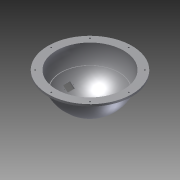
# Autodesk Inventor part: harvey_ballCup_ADNS9800_Vers1_1
Saved by Autodesk Inventor 2016 (Build 200138000, 138)
## iProperties
Created: 2012-05-12
Part Number: harvey_ballCup_ADNS9800_Vers1_1
Material: Generic
Document SubType Name: Modeling
Designer: charvey
Density: 1 g/cm^3
Appearance: Default
Author: charvey
Autodesk Inventor part; units mm, degrees
sketch "Sketch1" plane through (0, 0, 0) normal (0, 0, 1) x (1, 0, 0)
  arc A0 (0, -1.5875) -> (103.1875, 101.6) centre (0, 101.6) ccw
  arc A1 (0, -4.7625) -> (106.3625, 101.6) centre (0, 101.6) ccw
  line L0 (0, -1.5875) -> (0, -4.7625)
  line L1 (128.5875, 101.6) -> (128.5875, 95.25)
  line L2 (128.5875, 95.25) -> (106.1728, 95.25)
  line L3 (103.1875, 101.6) -> (128.5875, 101.6)
  arc A2 (0, 0) -> (87.9882, 50.8) centre (0, 101.6) ccw
  line L4 (87.9882, 50.8) -> (89.8166, 50.8)
  line L5 (0, 0) -> (0, -1.5875)
  dimension "d0" = 101.6
  dimension "d1" = 103.1875
  dimension "d2" = 106.3625
  dimension "d3" = 25.4
  dimension "d4" = 6.35
  dimension "d11" = 50.8
  constraints: 12 end point, 8 point on circle, 3 centre point, 2 coincident, 2 horizontal alignment, 2 parallel, 2 perpendicular, 1 point on line, 1 vertical
  measures "d0" distance of L5.start A0.centre
  measures "d1" distance of L0.start A0.centre
  measures "d2" distance of L0.end A1.centre
  measures "d3" distance of L3.start L1.start
  measures "d4" distance of L1.start L1.end
  measures "d11" vertical distance of L5.start L4.start
revolve "Revolution3" add sketch "Sketch1" angle 360 about axis through (0, -1.5875, 0) along (0, -1, 0)
ref_plane "Work Plane1" through (0, 127, 0) normal (0, 1, 0) x (-1, 0, 0)
sketch "Sketch4" plane through (0, 127, 0) normal (0, 1, 0) x (-1, 0, 0)
  line L0 (0, 0) -> (-141.4138, 0)
  line L1 (-141.4138, 0) -> (-141.4138, -141.6884)
  line L2 (-141.4138, -141.6884) -> (0, -141.6884)
  line L3 (0, -141.6884) -> (0, 0)
  constraints: 8 end point, 2 parallel, 1 horizontal, 1 perpendicular
sketch "Sketch13" plane through (0, 0, 0) normal (1, 0, 0) x (0, 1, 0)
  arc A0 (50.8, 87.9882) -> (50.8, -87.9882) centre (101.6, 0) ccw projected
  line L0 (50.8, 89.8166) -> (50.8, 87.9882) projected
  arc A1 (101.6, 103.1875) -> (50.8, 89.8166) centre (101.6, 0) ccw projected
  line L1 (101.6, -103.1875) -> (101.6, -128.5875) projected
  line L2 (101.6, -128.5875) -> (95.25, -128.5875) projected
  line L3 (95.25, -128.5875) -> (95.25, -106.1728) projected
  arc A2 (95.25, 106.1728) -> (95.25, -106.1728) centre (101.6, 0) ccw projected
  line L4 (50.8, -87.9882) -> (50.8, -89.8166) projected
  arc A3 (50.8, -89.8166) -> (101.6, -103.1875) centre (101.6, 0) ccw projected
  line L5 (95.25, 106.1728) -> (95.25, 128.5875) projected
  line L6 (95.25, 128.5875) -> (101.6, 128.5875) projected
  line L7 (101.6, 128.5875) -> (101.6, 103.1875) projected
  point P0 (0, 0)
  point P1 (4.2852, 29.1958)
  dimension "d18" = 16.7
  constraints: 1 coincident, 1 point on circle
hole "Hole2" at (0, 101.6, 0) direction (0, -0.9578, 0.2874) diameter 6.35 end through all
pattern_circular "Circular Pattern1" count 8 over 360 about axis through (0, 50.8, 0) along (0, -1, 0) of "Hole2"
ref_plane "Work Plane3" through (0, 203.2, 0) normal (0, 1, 0) x (-1, 0, 0)
sketch "Sketch14" plane through (0, 203.2, 0) normal (0, 1, 0) x (-1, 0, 0)
  circle A0 centre (0, 0) radius 128.5875 projected
  circle A1 centre (0, 0) radius 103.1875 projected
  point P0 (0, 119.0625)
  dimension "d41" = 119.0625
  constraints: 1 vertical alignment
  measures "d41" distance of point (0, 119.062) A0.centre
hole "Hole3" at (0, 203.2, 119.0625) direction (0, -1, 0) diameter 4.4958 end through all
pattern_circular "Circular Pattern2" count 8 over 360 about axis through (0, 50.8, 0) along (0, -1, 0) of "Hole3"
ref_plane "Work Plane4" through (0, -4.7625, 0) normal (0, 1, 0) x (-1, 0, 0)
sketch "Sketch15" plane through (0, -4.7625, 0) normal (0, 1, 0) x (-1, 0, 0)
  line L0 (0.0127, 0.0127) -> (-0.0127, 0.0127)
  line L1 (-0.0127, 0.0127) -> (-0.0127, -0.0127)
  line L2 (-0.0127, -0.0127) -> (0.0127, -0.0127)
  line L3 (0.0127, -0.0127) -> (0.0127, 0.0127)
  line L4 (0.0127, 0.0127) -> (-0.0127, -0.0127) construction
  line L5 (-0.0127, 0.0127) -> (0.0127, -0.0127) construction
  point P0 (0, 0)
  dimension "d52" = 0.0254
  dimension "d53" = 0.0254
  constraints: 12 end point, 2 midpoint, 2 parallel, 1 horizontal, 1 perpendicular
  measures "d52" distance of L2.end L1.end
  measures "d53" distance of L1.end L0.end
sketch "Sketch16" plane through (0, -4.7625, 0) normal (0, 1, 0) x (-1, 0, 0)
  line L0 (-0.0254, 0.0254) -> (0.0254, 0.0254)
  line L1 (0.0254, 0.0254) -> (0.0254, -0.0254)
  line L2 (0.0254, -0.0254) -> (-0.0254, -0.0254)
  line L3 (-0.0254, -0.0254) -> (-0.0254, 0.0254)
  line L4 (-0.0254, 0.0254) -> (0.0254, -0.0254) construction
  line L5 (0.0254, 0.0254) -> (-0.0254, -0.0254) construction
  point P0 (0, 0)
  dimension "d54" = 0.0508
  dimension "d55" = 0.0508
  constraints: 12 end point, 2 midpoint, 2 parallel, 1 horizontal, 1 perpendicular
  measures "d54" distance of L1.end L2.end
  measures "d55" distance of L0.end L1.end
extrude "Extrusion2" cut sketch "Sketch15" along normal through all
extrude "Extrusion3" cut sketch "Sketch16" along normal blind 3.175
ref_plane "Work Plane7" through (-68.3685, 20.1216, 0) normal (0.6428, 0.766, 0) x (-0.766, 0.6428, 0)
ref_plane "Work Plane6" through (-0.0127, -1.5875, -0.0063) normal (0.6428, 0.766, 0) x (0, 0, -1)
ref_plane "Work Plane9" through (0, 20.1216, 68.3685) normal (0, 0.766, -0.6428) x (-1, 0, 0)
ref_plane "Work Plane8" through (-0.0063, -1.5875, 0.0127) normal (0, 0.766, -0.6428) x (-1, 0, 0)
sketch "Sketch17" plane through (-68.3685, 20.1216, 0) normal (0.6428, 0.766, 0) x (-0.766, 0.6428, 0)
  line L0 (4.699, -5.842) -> (-4.699, -5.842)
  line L1 (-4.699, -5.842) -> (-4.699, 5.842)
  line L2 (-4.699, 5.842) -> (4.699, 5.842)
  line L3 (4.699, 5.842) -> (4.699, -5.842)
  line L4 (4.699, -5.842) -> (-4.699, 5.842) construction
  line L5 (-4.699, -5.842) -> (4.699, 5.842) construction
  point P0 (-65.3072, 0)
  point P1 (0, 0)
  dimension "d62" = 9.398
  dimension "d63" = 11.684
  constraints: 12 end point, 2 midpoint, 2 parallel, 1 horizontal, 1 perpendicular
  measures "d62" distance of L1.end L2.end
  measures "d63" distance of L0.end L1.end
sketch "Sketch18" plane through (-68.3685, 20.1216, 0) normal (0.6428, 0.766, 0) x (-0.766, 0.6428, 0)
  line L0 (9.525, -10.668) -> (-9.525, -10.668)
  line L1 (-9.525, -10.668) -> (-9.525, 10.668)
  line L2 (-9.525, 10.668) -> (9.525, 10.668)
  line L3 (9.525, 10.668) -> (9.525, -10.668)
  line L4 (9.525, -10.668) -> (-9.525, 10.668) construction
  line L5 (-9.525, -10.668) -> (9.525, 10.668) construction
  point P0 (-65.3072, 0)
  point P1 (0, 0)
  dimension "d64" = 19.05
  dimension "d65" = 21.336
  constraints: 12 end point, 2 midpoint, 2 parallel, 1 horizontal, 1 perpendicular
  measures "d64" distance of L1.end L2.end
  measures "d65" distance of L0.end L1.end
extrude "Extrusion4" cut sketch "Sketch17" along normal through all
extrude "Extrusion5" cut sketch "Sketch18" along normal through all
sketch "Sketch19" plane through (0, 20.1216, 68.3685) normal (0, 0.766, -0.6428) x (-1, 0, 0)
  line L0 (5.842, 4.699) -> (-5.842, 4.699)
  line L1 (-5.842, 4.699) -> (-5.842, -4.699)
  line L2 (-5.842, -4.699) -> (5.842, -4.699)
  line L3 (5.842, -4.699) -> (5.842, 4.699)
  line L4 (5.842, 4.699) -> (-5.842, -4.699) construction
  line L5 (-5.842, 4.699) -> (5.842, -4.699) construction
  point P0 (0, -65.3072)
  point P1 (0, 0)
  dimension "d70" = 11.684
  dimension "d71" = 9.398
  constraints: 12 end point, 2 midpoint, 2 parallel, 1 horizontal, 1 perpendicular
  measures "d70" distance of L2.end L1.end
  measures "d71" distance of L1.end L0.end
extrude "Extrusion6" cut sketch "Sketch19" along normal through all
sketch "Sketch20" plane through (0, 20.1216, 68.3685) normal (0, 0.766, -0.6428) x (-1, 0, 0)
  line L0 (10.668, 9.525) -> (-10.668, 9.525)
  line L1 (-10.668, 9.525) -> (-10.668, -9.525)
  line L2 (-10.668, -9.525) -> (10.668, -9.525)
  line L3 (10.668, -9.525) -> (10.668, 9.525)
  line L4 (10.668, 9.525) -> (-10.668, -9.525) construction
  line L5 (-10.668, 9.525) -> (10.668, -9.525) construction
  point P0 (0, -65.3072)
  point P1 (0, 0)
  dimension "d74" = 21.336
  dimension "d75" = 19.05
  constraints: 12 end point, 2 midpoint, 2 parallel, 1 horizontal, 1 perpendicular
  measures "d74" distance of L2.end L1.end
  measures "d75" distance of L1.end L0.end
extrude "Extrusion7" cut sketch "Sketch20" along normal through all
sketch "Sketch21" plane through (0, 20.1216, 68.3685) normal (0, 0.766, -0.6428) x (-1, 0, 0)
  circle A0 centre (0, 0) radius 17.78
  point P0 (0, -65.3072)
  dimension "d78" = 35.56
  constraints: 1 centre point
  measures "d78" diameter of A0
extrude "Extrusion8" cut sketch "Sketch21" along normal blind 1.5875
sketch "Sketch22" plane through (-68.3685, 20.1216, 0) normal (0.6428, 0.766, 0) x (-0.766, 0.6428, 0)
  circle A0 centre (0, 0) radius 17.78
  point P0 (-65.3072, 0)
  dimension "d81" = 35.56
  constraints: 1 centre point
  measures "d81" diameter of A0
extrude "Extrusion9" cut sketch "Sketch22" along normal blind 1.5875
sketch "Sketch23" plane through (-68.3685, 20.1216, 0) normal (0.6428, 0.766, 0) x (-0.766, 0.6428, 0)
  line L0 (9.525, 10.668) -> (9.525, -10.668)
  arc A0 (9.525, -10.668) -> (9.525, 10.668) centre (5.4215, 0) ccw
  point P0 (-65.3072, 0)
  dimension "d87" = 21.336
  dimension "d88" = 11.43
  constraints: 2 end point, 2 point on circle, 1 centre point, 1 vertical
  measures "d87" distance of L0.start L0.end
  measures "d88" radius of A0
extrude "Extrusion10" cut sketch "Sketch23" along normal blind 3.175
sketch "Sketch24" plane through (0, 20.1216, 68.3685) normal (0, 0.766, -0.6428) x (-1, 0, 0)
  line L0 (10.668, 9.525) -> (-10.668, 9.525)
  arc A0 (10.668, 9.525) -> (-10.668, 9.525) centre (0, 5.4215) ccw
  point P0 (0, -65.3072)
  dimension "d89" = 21.336
  dimension "d90" = 11.43
  constraints: 2 end point, 2 point on circle, 1 centre point, 1 horizontal
  measures "d89" distance of L0.start L0.end
  measures "d90" radius of A0
extrude "Extrusion11" cut sketch "Sketch24" along normal blind 3.175
sketch "Sketch29" plane through (-68.3685, 20.1216, 0) normal (0.6428, 0.766, 0) x (-0.766, 0.6428, 0)
  circle A0 centre (0, 13.8963) radius 0.889
  circle A1 centre (0, -13.3883) radius 0.889
  point P0 (-65.3072, 0)
  dimension "d116" = 1.778
  dimension "d117" = 1.778
  constraints: 2 centre point
  measures "d116" diameter of A0
  measures "d117" diameter of A1
extrude "Extrusion13" cut sketch "Sketch29" along normal through all
sketch "Sketch30" plane through (0, 20.1216, 68.3685) normal (0, 0.766, -0.6428) x (-1, 0, 0)
  circle A0 centre (13.3883, 0) radius 0.889
  circle A1 centre (-13.3883, 0) radius 0.889
  point P0 (0, -65.3072)
  dimension "d120" = 1.778
  dimension "d121" = 1.778
  constraints: 2 centre point
  measures "d120" diameter of A0
  measures "d121" diameter of A1
extrude "Extrusion14" cut sketch "Sketch30" along normal through all
body "Solid2"
